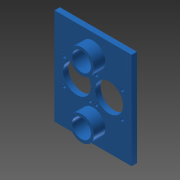
# Autodesk Inventor part: XCarriageV9Top
Saved by Autodesk Inventor 2015 (Build 190159000, 159)
## iProperties
Created: 2014-08-22
Part Number: XCarriageV9Top
Material: ABS Plastic
Document SubType Name: Modeling
Designer: Jack
Density: 1.06 g/cm^3
Appearance: Cyan
Author: Jack
Autodesk Inventor part; units mm, degrees
ref_plane "YZ Plane" through (0, 0, 0) normal (1, 0, 0) x (0, 1, 0)
ref_plane "XZ Plane" through (0, 0, 0) normal (0, 1, 0) x (-1, 0, 0)
ref_plane "XY Plane" through (0, 0, 0) normal (0, 0, 1) x (1, 0, 0)
sketch "Sketch1" plane through (0, 0, 0) normal (0, 1, 0) x (-1, 0, 0)
  line L0 (0, 0) -> (72, 0)
  line L1 (72, 0) -> (72, -90)
  line L2 (72, -90) -> (0, -90)
  line L3 (0, -90) -> (0, 0)
  dimension "d0" = 72
  dimension "d1" = 90
  constraints: 8 end point, 2 parallel, 1 horizontal, 1 perpendicular
  measures "d0" distance of L0.start L0.end
  measures "d1" distance of L2.end L0.start
extrude "Extrusion1" add sketch "Sketch1" along normal blind 5
sketch "Sketch2" plane through (0, 0, 0) normal (0, -1, 0) x (1, 0, 0)
  line L0 (-72, 0) -> (-72, -90) projected
  line L1 (-72, -90) -> (0, -90) projected
  circle A0 centre (-36, -72) radius 8.75
  circle A1 centre (-36, -18) radius 8.75
  circle A2 centre (-36, -18) radius 11.5
  circle A3 centre (-36, -72) radius 11.5
  dimension "d4" = 17.5
  dimension "d5" = 23
  dimension "d6" = 54
  dimension "d7" = 18
  dimension "d8" = 36
  constraints: 4 centre point, 2 coincident, 2 equal radius, 1 vertical alignment
  measures "d4" diameter of A1
  measures "d5" diameter of A2
  measures "d6" distance of A0.centre A1.centre
  measures "d7" distance from line of L1 A0.centre
  measures "d8" distance from line of L0 A0.centre
extrude "Extrusion2" add sketch "Sketch2" along normal blind 10.7
sketch "Sketch3" plane through (-36, 0, -18) normal (0, -1, 0) x (1, 0, 0)
  circle A0 centre (0, 0) radius 8.75 projected
  circle A1 centre (0, -54) radius 8.75 projected
  point P0 (36, 18)
extrude "Extrusion3" cut sketch "Sketch3" against normal up to surface (5 mm away)
sketch "Sketch4" plane through (0, 0, 0) normal (0, -1, 0) x (1, 0, 0)
  line L0 (0, 0) -> (-72, 0) projected
  line L1 (-72, 0) -> (-72, -90) projected
  line L2 (0, -90) -> (0, 0) projected
  circle A0 centre (-21, -45) radius 13
  circle A1 centre (-51, -45) radius 13
  dimension "d14" = 26
  dimension "d16" = 21
  dimension "d17" = 21
  dimension "d18" = 45
  constraints: 2 centre point, 1 equal radius, 1 horizontal alignment
  measures "d14" diameter of A1
  measures "d16" distance from line of L1 A1.centre
  measures "d17" distance from line of L2 A0.centre
  measures "d18" distance from line of L0 A0.centre
extrude "Extrusion4" cut sketch "Sketch4" against normal up to surface (5 mm away)
sketch "Sketch5" plane through (0, 0, 0) normal (0, -1, 0) x (1, 0, 0)
  circle A0 centre (-21, -45) radius 13 projected
  circle A1 centre (-51, -45) radius 13 projected
  circle A2 centre (-9, -57) radius 1.5
  circle A3 centre (-9, -33) radius 1.5
  circle A4 centre (-33, -57) radius 1.5
  circle A5 centre (-33, -33) radius 1.5
  circle A6 centre (-39, -33) radius 1.5
  circle A7 centre (-39, -57) radius 1.5
  circle A8 centre (-63, -57) radius 1.5
  circle A9 centre (-63, -33) radius 1.5
  dimension "d21" = 3
  dimension "d22" = 24
  dimension "d23" = 24
  dimension "d24" = 24
  dimension "d25" = 12
  dimension "d26" = 12
  dimension "d27" = 12
  constraints: 8 centre point, 7 equal radius, 6 horizontal alignment, 4 vertical alignment
  measures "d21" diameter of A2
  measures "d22" distance of A8.centre A7.centre
  measures "d23" distance of A2.centre A4.centre
  measures "d24" distance of A2.centre A3.centre
  measures "d25" horizontal distance of A0.centre A2.centre
  measures "d26" horizontal distance of A0.centre A2.centre
  measures "d27" horizontal distance of A1.centre A7.centre
extrude "Extrusion5" cut sketch "Sketch5" against normal up to surface (5 mm away) contours A2 | A3 | A4 | A5 | A6 | A7 | A8 | A9
body "Solid1"
